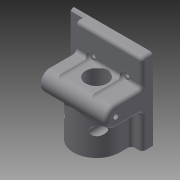
# Autodesk Inventor part: Carraige
Saved by Autodesk Inventor 2015 SP1 (Build 190203100, 203)
## iProperties
Created: 2015-02-03
Part Number: Carraige
Material: Generic
Document SubType Name: Modeling
Designer: Joseph
Density: 1 g/cm^3
Appearance: Default
Author: Joseph
Autodesk Inventor part; units mm, degrees
ref_plane "YZ Plane" through (0, 0, 0) normal (1, 0, 0) x (0, 1, 0)
ref_plane "XZ Plane" through (0, 0, 0) normal (0, 1, 0) x (-1, 0, 0)
ref_plane "XY Plane" through (0, 0, 0) normal (0, 0, 1) x (1, 0, 0)
sketch "Sketch1" plane through (0, 0, 0) normal (0, 0, 1) x (1, 0, 0)
  line L0 (0, 0) -> (0, 48) construction
  line L1 (0, 0) -> (27, 0) construction
  line L2 (27, 0) -> (27, 48) construction
  line L3 (0, 48) -> (27, 48) construction
  line L4 (33.5, 48) -> (-6.5, 48)
  line L5 (-6.5, 48) -> (-6.5, 0)
  line L6 (-6.5, 0) -> (33.5, 0)
  line L7 (33.5, 0) -> (33.5, 48)
  line L8 (33.5, 48) -> (-6.5, 0) construction
  line L9 (-6.5, 48) -> (33.5, 0) construction
  point P0 (13.5, 24)
  dimension "d0" = 40
  constraints: 12 end point, 2 midpoint, 2 parallel, 1 horizontal, 1 perpendicular
  measures "d0" distance of L6.end L5.end
extrude "Extrusion1" add sketch "Sketch1" along normal blind 30
sketch "Sketch5" plane through (-6.5, 0, 0) normal (-1, 0, 0) x (0, 0, 1)
  line L0 (0, 48) -> (0, 0) projected
  line L1 (0, 0) -> (30, 0) projected
  arc A0 (21.9437, 20.0563) -> (21.9437, 32.0563) centre (21.9437, 26.0563) ccw
  line L2 (0, 48) -> (4.4156, 48)
  line L3 (6.4156, 0) -> (0, 0)
  line L4 (0, 0) -> (0, 48)
  line L5 (21.9437, 32.0563) -> (8.4156, 32.0563)
  line L6 (8.4156, 20.0563) -> (21.9437, 20.0563)
  line L7 (6.4156, 46) -> (6.4156, 34.0563)
  line L8 (6.4156, 18.0563) -> (6.4156, 0)
  arc A1 (6.4156, 34.0563) -> (8.4156, 32.0563) centre (8.4156, 34.0563) ccw
  arc A2 (8.4156, 20.0563) -> (6.4156, 18.0563) centre (8.4156, 18.0563) ccw
  arc A3 (6.4156, 46) -> (4.4156, 48) centre (4.4156, 46) ccw
  dimension "d19" = 2
  dimension "d20" = 2
  dimension "d37" = 6
  constraints: 14 end point, 8 point on circle, 6 tangent, 4 centre point, 4 parallel, 2 horizontal, 2 perpendicular, 1 equal radius, 1 point on line
  measures "d19" radius of A1
  measures "d20" radius of A3
  measures "d37" radius of A0
extrude "Extrusion5" cut sketch "Sketch5" against normal through all keep common part
sketch "Sketch6" plane through (-6.5, 0, 0) normal (0, -1, 0) x (1, 0, 0)
  line L0 (6.5, -10) -> (6.5, 0) construction
  line L1 (33.5, 0) -> (33.5, -10) construction
  line L2 (6.5, 0) -> (33.5008, 0)
  line L3 (33.5008, 0) -> (33.5008, 13.4489)
  line L4 (6.5, 16.4625) -> (6.5, 0)
  arc A0 (33.5008, 13.4489) -> (6.5, 16.4625) centre (19.8322, 13.4489) ccw
  circle A1 centre (19.8322, 13.4489) radius 6.5
  line L5 (19.8322, 13.4489) -> (20.0004, 0) construction
  point P0 (19.8322, 27.1175)
  dimension "d23" = 13
  dimension "d24" = 13.45
  constraints: 8 end point, 3 point on circle, 2 centre point, 1 coincident, 1 horizontal, 1 midpoint, 1 parallel, 1 perpendicular, 1 tangent
  measures "d23" diameter of A1
  measures "d24" distance of L5.start L5.end
extrude "Extrusion6" add sketch "Sketch6" against normal up to next
sketch "Sketch2" plane through (-6.5, 0, 0) normal (-1, 0, 0) x (0, 0, 1)
  line L0 (0, 48) -> (0, 0) projected
  circle A0 centre (21.9437, 26.0563) radius 1.5
  line L1 (-3.5, 32.7705) -> (0, 32.7705) construction
  line L2 (-3.5, 15.2295) -> (0, 15.2295) construction
  line L3 (0, 32.7705) -> (0, 15.2295) construction
  line L4 (0, 52.771) -> (2, 52.771) construction
  line L5 (2, 52.771) -> (2, -5.2729) construction
  line L6 (2, -5.2729) -> (0, -5.2729) construction
  line L7 (0, -5.2729) -> (0, 52.771) construction
  line L8 (2, 49.5092) -> (13, 49.5092) construction
  line L9 (13, 49.5092) -> (13, -2.3456) construction
  line L10 (13, -2.3456) -> (2, -2.3456) construction
  line L11 (2, -2.3456) -> (2, 49.5092) construction
  line L12 (21.9437, 20.0563) -> (8.4156, 20.0563)
  arc A1 (21.9437, 20.0563) -> (21.9437, 32.0563) centre (21.9437, 26.0563) ccw projected
  dimension "d3" = 3
  dimension "d14" = 2
  dimension "d15" = 11
  constraints: 24 end point, 4 horizontal, 4 parallel, 2 perpendicular, 1 centre point, 1 coincident, 1 collinear, 1 point on line, 4 other
  measures "d3" diameter of A0
  measures "d14" distance of L5.end L6.end
  measures "d15" distance of L9.end L10.end
extrude "Extrusion2" cut sketch "Sketch2" against normal through all
sketch "Sketch3" plane through (-6.5, 0, 0) normal (-1, 0, 0) x (0, 0, 1)
  line L0 (0, 0) -> (30, 0) projected
  line L1 (0, 48) -> (1, 48)
  line L2 (2, 47) -> (2, 1)
  line L3 (1, 0) -> (0, 0)
  line L4 (0, 0) -> (0, 48)
  line L5 (1, 48) -> (2, 47)
  line L6 (2, 1) -> (1, 0)
  point P0 (2, 0)
  point P1 (2, 48)
  dimension "d7" = 2
  dimension "d8" = 1
  dimension "d9" = 1
  dimension "d10" = 1
  dimension "d11" = 1
  constraints: 12 end point, 5 point on line, 2 parallel, 1 horizontal, 1 perpendicular
  measures "d7" distance of point (2, 0) L3.end
  measures "d8" distance of L1.end point (2, 48)
  measures "d9" distance of L2.start point (2, 48)
  measures "d10" distance of L2.end point (2, 0)
  measures "d11" distance of L3.start point (2, 0)
extrude "Extrusion3" add sketch "Sketch3" along normal blind 7
sketch "Sketch7" plane through (33.5, 0, 0) normal (0, -1, 0) x (1, 0, 0)
  circle A0 centre (-20.1678, 13.4489) radius 6.5 projected
  arc A1 (-6.4992, 13.4489) -> (-33.5, 16.4625) centre (-20.1678, 13.4489) ccw projected
  circle A2 centre (-20.1678, 13.4489) radius 6.5
  point P0 (-33.5, 0)
  constraints: 1 centre point, 1 coincident, 1 concentric
extrude "Extrusion7" cut sketch "Sketch7" against normal through all
fillet "Fillet1" radius 2 27 edges at (26.2395, 20.0563, 17.9468) (27.0008, 20.0563, 10.9323) (27.0008, 19.4705, 7.0014) (27.0008, 9.0282, 6.4156) (13.3366, 23.0179, 27.1175) (1.0035, 20.0563, 19.3508) (0, 20.0563, 12.439) (0, 19.4705, 7.0014) (0, 9.0282, 6.4156) (33.5, 26.0563, 27.9437) (33.5, 32.0563, 15.1796) (33.5, 32.6421, 7.0014) (33.5, 40.0282, 6.4156) (33.5, 47.4142, 5.8298) (33.5, 48, 2.2078) (33.5, 19.4705, 7.0014) (33.5, 9.0282, 6.4156) (33.5, 20.0563, 15.1796) (-6.5, 20.0563, 15.1796) (-6.5, 19.4705, 7.0014) (-6.5, 9.0282, 6.4156) (-6.5, 32.0563, 15.1796) (-6.5, 32.6421, 7.0014) (-6.5, 40.0282, 6.4156) (-6.5, 47.4142, 5.8298) (-6.5, 48, 2.7078) (-6.5, 26.0563, 27.9437)
ref_plane "Work Plane1" through (-6.5, 26.0563, 27.9437) normal (0, 0, -1) x (-1, 0, 0)
sketch "Sketch8" plane through (-6.5, 26.0563, 27.9437) normal (0, 0, -1) x (-1, 0, 0)
  circle A0 centre (-9.5814, 7.9437) radius 1.2295 construction
  circle A1 centre (-29.5814, 7.9437) radius 1.2295 construction
  circle A2 centre (-29.5814, -12.0563) radius 1.2295 construction
  circle A3 centre (-9.5814, -12.0563) radius 1.2295 construction
  point P0 (-6.5, -26.0563)
  constraints: 4 coincident
hole "Hole1" at (3.0814, 34, 27.9437) at (23.0814, 34, 27.9437) at (23.0814, 14, 27.9437) at (3.0814, 14, 27.9437) direction (0, 0, -1) diameter 3 end through all counterbore diameter 5.5 counterbore depth 23 clearance for "Socket Head Cap Screw" size "M2.5" standard "Ansi Metric M Profile"
sketch "Sketch9" plane through (-13.5, 0, 0) normal (0, -1, 0) x (1, 0, 0)
  arc A0 (40.5008, 13.4489) -> (13.5, 16.4625) centre (26.8322, 13.4489) ccw projected
  circle A1 centre (21.1466, 6.0618) radius 1.2295 construction
  circle A2 centre (23.0749, 21.9452) radius 1.2295 construction
  circle A3 centre (35.8662, 12.3335) radius 1.2295 construction
  circle A4 centre (26.8322, 13.4489) radius 9.29 construction
  line L0 (26.8322, 22.7389) -> (18.7869, 8.804) construction
  line L1 (34.8776, 8.804) -> (18.7869, 8.804) construction
  line L2 (34.8776, 8.804) -> (26.8322, 22.7389) construction
  point P0 (13.5, 0)
  constraints: 6 end point, 4 coincident, 4 point on circle, 2 equal length, 1 centre point, 1 horizontal
hole "Hole2" at (13.3322, 0, 22.7389) at (5.2869, 0, 8.804) at (21.3776, 0, 8.804) direction (0, 1, 0) diameter 2.459 depth 8.8 tip angle 118 thread size "M3x0.5" class "6H" standard "ANSI Metric M Profile"
equation "\"d9\" = d8"
equation "\"d10\" = d8"
equation "\"d11\" = d10"
body "Solid1"
